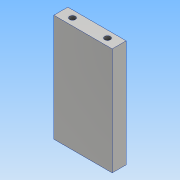
# Autodesk Inventor part: Top_Separator Block
Saved by Autodesk Inventor 2018.1 (Build 221171000, 171)
## iProperties
Created: 2019-03-20
Part Number: Top_Separator Block
Material: Aluminum 6061
Document SubType Name: Modeling
Designer: James
Density: 2.7 g/cm^3
Appearance: Aluminum - Flat
Author: James
Autodesk Inventor part; units mm, degrees
ref_plane "YZ Plane" through (0, 0, 0) normal (1, 0, 0) x (0, 1, 0)
ref_plane "XZ Plane" through (0, 0, 0) normal (0, 1, 0) x (-1, 0, 0)
ref_plane "XY Plane" through (0, 0, 0) normal (0, 0, 1) x (1, 0, 0)
sketch "Sketch1" plane through (0, 0, 0) normal (0, 1, 0) x (-1, 0, 0)
  line L0 (0, 0) -> (25, 0)
  line L1 (25, 0) -> (25, -46)
  line L2 (25, -46) -> (0, -46)
  line L3 (0, -46) -> (0, 0)
  dimension "d0" = 25
  dimension "d1" = 46
  constraints: 8 end point, 2 parallel, 1 horizontal, 1 perpendicular
  measures "d0" distance of L1.end L2.end
  measures "d1" distance of L0.end L1.end
extrude "Extrusion1" add sketch "Sketch1" along normal blind 6
sketch "Sketch2" plane through (-25, 0, 0) normal (0, 0, 1) x (1, 0, 0)
  line L0 (25, 0) -> (25, 6) projected
  line L1 (0, 0) -> (0, 6) projected
  point P0 (5, 3)
  point P1 (20, 3)
  point P2 (25, 3)
  point P3 (25, 3)
  dimension "d4" = 5
  dimension "d5" = 5
  dimension "d6" = 15
  constraints: 2 horizontal alignment, 2 midpoint
  measures "d4" distance from line of point (5, 3) L1
  measures "d5" distance from line of L0 point (20, 3)
  measures "d6" distance of point (20, 3) point (5, 3)
hole "Hole1" at (-20, 3, 0) at (-5, 3, 0) direction (0, 0, -1) diameter 2.459 depth 8.8 tip angle 118 thread size "M3x0.5" class "6H" standard "ANSI Metric M Profile"
ref_plane "Work Plane1" through (-25, 0, -23) normal (0, 0, 1) x (1, 0, 0)
mirror "Mirror1" about plane through (-25, 0, -23) normal (0, 0, 1) of "Hole1"
equation "\"d5\" = d4"
body "Solid1"
